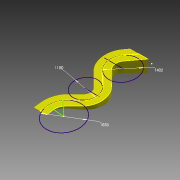
# Autodesk Inventor part: Down Hill_赤2
Saved by Autodesk Inventor 2015 (Build 190159000, 159)
## iProperties
Created: 2015-09-14
Part Number: Down Hill_赤2
Material: 一般
Document SubType Name: Modeling
Designer: nobuhiro
Density: 1 g/cm^3
Appearance: 滑らか - 黄
Author: nobuhiro
Autodesk Inventor part; units mm, degrees
ref_plane "YZ Plane" through (0, 0, 0) normal (1, 0, 0) x (0, 1, 0)
ref_plane "XZ Plane" through (0, 0, 0) normal (0, 1, 0) x (-1, 0, 0)
ref_plane "XY Plane" through (0, 0, 0) normal (0, 0, 1) x (1, 0, 0)
sketch "スケッチ1" plane through (0, 0, 0) normal (0, 0, 1) x (1, 0, 0)
  line L0 (1130.6278, 0) -> (1301.8139, -171.1861)
  line L1 (282.0996, 0) -> (877.5498, -595.4502)
  line L2 (1130.6278, 0) -> (282.0996, 0)
  circle A0 centre (594, -879) radius 1001 construction
  arc A1 (1296.7129, -1591.8784) -> (1296.7129, -1591.8784) centre (389.9346, -671.9826) ccw
  line L3 (1296.7129, -1591.8784) -> (686.4168, -2193.4718)
  circle A2 centre (890, -2400) radius 290 construction
  line L4 (713.3557, -2629.993) -> (1149.395, -2964.8896)
  line L5 (1595, -4169) -> (1595, -3869)
  circle A3 centre (455, -3869) radius 1140 construction
  arc A4 (875.5064, -1164.5786) -> (877.5498, -595.4502) centre (594, -879) ccw construction
  circle A5 centre (890, -2400) radius 890 construction
  circle A6 centre (455, -3869) radius 540 construction
  line L6 (783.9239, -3440.7372) -> (347.8846, -3105.8406)
  line L7 (265.2103, -1766.1721) -> (875.5064, -1164.5786)
  line L8 (995, -3869) -> (995, -4169)
  line L9 (995, -4169) -> (1595, -4169)
  arc A7 (1296.7129, -1591.8784) -> (1301.8139, -171.1861) centre (594, -879) ccw
  arc A8 (265.2103, -1766.1721) -> (347.8846, -3105.8406) centre (890, -2400) ccw
  arc A9 (686.4168, -2193.4718) -> (713.3557, -2629.993) centre (890, -2400) ccw
  arc A10 (875.5064, -1164.5786) -> (877.5498, -595.4502) centre (594, -879) ccw
  arc A11 (995, -3869) -> (783.9239, -3440.7372) centre (455, -3869) ccw
  arc A12 (1595, -3869) -> (1149.395, -2964.8896) centre (455, -3869) ccw
  line L10 (0, -4169) -> (1595, -4169) construction
  line L11 (1595, -4169) -> (1595, -4131.3008) construction
  line L12 (0, -4169) -> (0, 0) construction
  line L13 (0, 0) -> (1595, 0) construction
  line L14 (-1130.6278, 0) -> (-1301.8139, -171.1861)
  line L15 (-282.0996, 0) -> (-877.5498, -595.4502)
  line L16 (-1130.6278, 0) -> (-282.0996, 0)
  arc A13 (-1296.7129, -1591.8784) -> (-1296.7129, -1591.8784) centre (-389.9346, -671.9826) ccw
  line L17 (-1296.7129, -1591.8784) -> (-686.4168, -2193.4718)
  line L18 (-713.3557, -2629.993) -> (-1149.395, -2964.8896)
  line L19 (-1595, -4169) -> (-1595, -3869)
  line L20 (-783.9239, -3440.7372) -> (-347.8846, -3105.8406)
  line L21 (-265.2103, -1766.1721) -> (-875.5064, -1164.5786)
  line L22 (-995, -3869) -> (-995, -4169)
  line L23 (-995, -4169) -> (-1595, -4169)
  arc A14 (-1301.8139, -171.1861) -> (-1296.7129, -1591.8784) centre (-594, -879) ccw
  arc A15 (-347.8846, -3105.8406) -> (-265.2103, -1766.1721) centre (-890, -2400) ccw
  arc A16 (-713.3557, -2629.993) -> (-686.4168, -2193.4718) centre (-890, -2400) ccw
  arc A17 (-877.5498, -595.4502) -> (-875.5064, -1164.5786) centre (-594, -879) ccw
  arc A18 (-783.9239, -3440.7372) -> (-995, -3869) centre (-455, -3869) ccw
  arc A19 (-1149.395, -2964.8896) -> (-1595, -3869) centre (-455, -3869) ccw
  line L24 (0, -4169) -> (-1595, -4169) construction
  line L25 (-1595, -4169) -> (-1595, -4131.3008) construction
  line L26 (1595, -4169) -> (1595, 0) construction
  arc A20 (1120.2352, -2943.2235) -> (532.7643, -2869.5558) centre (890, -2400) ccw
  arc A21 (1086.1097, -1378.2285) -> (1089.6819, -383.3181) centre (594, -879) ccw
  line L27 (332.9203, 373.4434) -> (1089.6819, -383.3181)
  line L28 (475.8136, -1979.822) -> (1086.1097, -1378.2285)
  arc A22 (1295, -3933.8556) -> (965.1205, -3198.4902) centre (455, -3869) ccw
  line L29 (1295, -4169) -> (1295, -3933.8556)
  line L30 (965.1205, -3198.4902) -> (532.7643, -2869.5558)
  dimension "d1" = 1080
  dimension "d2" = 2280
  dimension "d3" = 580
  dimension "d4" = 1780
  dimension "d5" = 802
  dimension "d6" = 2002
  dimension "d16" = 45
  dimension "d19" = 1140
  dimension "d20" = 4169
  dimension "d21" = 0
  dimension "d22" = 600
  dimension "d35" = 3290
  dimension "d36" = 1769
  dimension "d37" = 300
  dimension "d39" = 300
  dimension "d41" = 1595
  dimension "d43" = 1001
  dimension "d55" = 1180
  dimension "d58" = 1402
  dimension "d59" = 300
  dimension "d60" = 1685
  dimension "d61" = 300
  constraints: 62 end point, 49 point on circle, 26 symmetric about line, 23 centre point, 20 tangent, 4 horizontal, 3 coincident, 3 parallel, 2 concentric, 2 perpendicular, 2 point on line, 1 collinear, 1 vertical, 7 other
  measures "d1" diameter of A6
  measures "d2" diameter of A3
  measures "d3" diameter of A2
  measures "d4" diameter of A5
  measures "d5" diameter of A4
  measures "d6" diameter of A0
  measures "d16" angle of L13 L1
  measures "d19" distance from line of A6.centre L11
  measures "d20" distance between parallel lines of L13 L10
  measures "d21" distance between parallel lines of L11 L5
  measures "d22" distance of L8.end L5.start
  measures "d35" distance from line of L10 A0.centre
  measures "d36" distance from line of L10 A5.centre
  measures "d37" distance from line of L10 A3.centre
  measures "d39" distance from line of L10 A6.centre
  measures "d41" distance between parallel lines of L12 L26
  measures "d43" distance from line of L26 A4.centre
  measures "d55" diameter of A20
  measures "d58" diameter of A21
  measures "d59" distance between parallel lines of L27 L1
  measures "d60" diameter of A22
  measures "d61" distance from line of L5.start L29
extrude "押し出し1" add sketch "スケッチ1" along normal blind 600 contours L16 L15 A17 A1 | A1 A17 L21 A15 A13 A14 L14 L16 | A13 A15 L20 A18 L22 L23 L19 A19 L18 A16 L17 | L21 A15 A1
sketch "スケッチ2" plane through (0, 0, 0) normal (1, 0, 0) x (0, 1, 0)
  line L0 (0, 0) -> (0, 600)
  line L1 (0, 600) -> (-4169, 0)
  line L2 (-4169, 0) -> (0, 0)
  dimension "d26" = 600
  dimension "d27" = 4169
  constraints: 6 end point, 1 perpendicular, 1 vertical
  measures "d26" distance of L0.start L0.end
  measures "d27" distance of L1.end L0.start
extrude "押し出し2" cut sketch "スケッチ2" along normal through all both and the other way through all keep common part
sketch "スケッチ3" plane through (-1130.6278, 0, 600) normal (0, -0.1424517, 0.9898018) x (1, 0, 0)
  line L0 (0, 0) -> (-171.1861, -172.9499) projected
  ellipse E0 centre (536.6278, -888.0566) end of major axis (536.6278, 123.257) minor radius 1001 (-171.1861, -172.9499) -> (-166.0851, -1608.28) ccw projected
  line L1 (-166.0851, -1608.28) -> (444.2109, -2216.0718) projected
  ellipse E1 centre (240.6278, -2424.728) end of major axis (240.6278, -2131.74) minor radius 290 (417.2721, -2657.0907) -> (444.2109, -2216.0718) ccw projected
  line L2 (417.2721, -2657.0907) -> (-18.7672, -2995.4378) projected
  ellipse E2 centre (675.6278, -3908.8635) end of major axis (675.6278, -2757.1178) minor radius 1140 (-18.7672, -2995.4378) -> (-464.3722, -3908.8635) ccw projected
  line L3 (-464.3722, -3908.8635) -> (-464.3722, -4211.9545) projected
  line L4 (-464.3722, -4211.9545) -> (135.6278, -4211.9545) projected
  line L5 (135.6278, -4211.9545) -> (135.6278, -3908.8635) projected
  ellipse E3 centre (675.6278, -3908.8635) end of major axis (675.6278, -4454.4273) minor radius 540 (346.7038, -3476.1882) -> (135.6278, -3908.8635) ccw projected
  line L6 (346.7038, -3476.1882) -> (782.7431, -3137.841) projected
  ellipse E4 centre (240.6278, -2424.728) end of major axis (240.6278, -3323.8979) minor radius 890 (782.7431, -3137.841) -> (865.4175, -1784.3695) ccw projected
  line L7 (865.4175, -1784.3695) -> (255.1214, -1176.5777) projected
  ellipse E5 centre (536.6278, -888.0566) end of major axis (536.6278, -1293.1882) minor radius 401 (253.078, -601.5853) -> (255.1214, -1176.5777) ccw projected
  line L8 (253.078, -601.5853) -> (848.5281, 0) projected
  line L9 (848.5281, 0) -> (0, 0) projected
  line L10 (32.4595, -374.5187) -> (119.5473, -286.5336)
  line L11 (119.5473, -286.5336) -> (161.7579, -286.5336)
  line L12 (161.7579, -286.5336) -> (49.4323, -400.0165)
  line L13 (52.9285, -1379.6036) -> (663.2246, -1987.3955)
  line L14 (607.0857, -2911.4653) -> (171.0464, -3249.8125)
  line L15 (-150.9058, -3908.8635) -> (-150.9058, -3925.4209)
  line L16 (-150.9058, -3925.4209) -> (-177.8386, -3925.4209)
  line L17 (-177.8386, -3925.4209) -> (-177.8386, -3908.8635)
  line L18 (156.8903, -3221.8135) -> (592.9296, -2883.4664)
  line L19 (646.4038, -2013.0459) -> (36.1077, -1405.254)
  line L20 (-177.8386, -3925.4209) -> (-177.8386, -4211.9545)
  line L21 (-150.9058, -3925.4209) -> (-150.9058, -4211.9545)
  line L22 (119.5473, -286.5336) -> (403.1588, 0)
  line L23 (161.7579, -286.5336) -> (445.3694, 0)
  line L24 (135.6278, -4196.9545) -> (-464.3722, -4196.9545)
  spline S0 degree 5 poles (49.4323, -400.0165) (6.0772, -443.8184) (-32.3846, -492.4635) (-65.2456, -545.2099) (-132.8167, -686.6868) (-159.1151, -842.5379) (-158.774, -938.5796) (-131.3678, -1094.2411) (-62.7886, -1235.2334) (-29.5508, -1287.7445) (9.2593, -1336.1136) (52.9285, -1379.6037) knots 0 0 0 0 0 0 0.283408 0.283408 0.283408 0.716588 0.716588 0.716588 1 1 1 1 1 1
  spline S1 degree 5 poles (663.2246, -1987.3955) (689.0757, -2013.1406) (712.9955, -2040.8251) (734.7988, -2070.2469) (790.8712, -2159.0366) (827.2909, -2258.2936) (841.914, -2325.8413) (852.2743, -2463.1111) (825.3116, -2598.1007) (802.6182, -2663.2752) (754.4609, -2757.1689) (688.0629, -2838.2566) (662.8873, -2864.7026) (635.8251, -2889.1648) (607.0856, -2911.4653) knots 0 0 0 0 0 0 0.174362 0.174362 0.174362 0.5005 0.5005 0.5005 0.826151 0.826151 0.826151 1 1 1 1 1 1
  spline S2 degree 5 poles (171.0463, -3249.8125) (111.0424, -3296.3728) (56.3825, -3349.8197) (8.1044, -3409.3151) (-74.0223, -3538.2511) (-125.0897, -3682.3398) (-142.3005, -3756.981) (-150.9059, -3832.9223) (-150.9059, -3908.8635) knots 0 0 0 0 0 0 0.500027 0.500027 0.500027 1 1 1 1 1 1
  spline S3 degree 5 poles (-177.8386, -3908.8635) (-177.8386, -3829.4629) (-168.8535, -3750.0621) (-150.8837, -3672.0169) (-97.7184, -3521.8667) (-12.2191, -3387.4922) (37.8624, -3325.6829) (94.5891, -3270.1564) (156.8903, -3221.8135) knots 0 0 0 0 0 0 0.501717 0.501717 0.501717 1 1 1 1 1 1
  spline S4 degree 5 poles (592.9296, -2883.4664) (637.1161, -2849.1796) (677.1472, -2809.5378) (712.1687, -2765.2259) (786.2835, -2643.7028) (821.3073, -2504.3486) (826.6322, -2417.1494) (808.8484, -2274.6041) (750.1598, -2144.9634) (720.8492, -2096.7232) (686.0109, -2052.4905) (646.4039, -2013.0458) knots 0 0 0 0 0 0 0.283586 0.283586 0.283586 0.71657 0.71657 0.71657 1 1 1 1 1 1
  spline S5 degree 5 poles (36.1078, -1405.254) (7.8648, -1377.1269) (-18.4304, -1347.0438) (-42.6049, -1315.1925) (-105.4626, -1219.3372) (-148.7354, -1112.4732) (-167.8679, -1039.6342) (-187.2712, -890.6974) (-168.9256, -741.6264) (-150.3095, -668.6481) (-107.7943, -561.4682) (-45.6173, -465.1561) (-21.6678, -433.1277) (4.4149, -402.8522) (32.4595, -374.5187) knots 0 0 0 0 0 0 0.174265 0.174265 0.174265 0.499975 0.499975 0.499975 0.825708 0.825708 0.825708 1 1 1 1 1 1
  point P0 (1130.6278, -85.471)
  dimension "d31" = 30
  dimension "d32" = 15
  constraints: 30 end point, 11 parallel, 6 point on line, 2 collinear, 2 perpendicular, 1 vertical, 28 other
  measures "d31" distance between parallel lines of L12 L10
  measures "d32" distance between parallel lines of L4 L24
extrude "押し出し3" add sketch "スケッチ3" along normal blind 0.1 contours L9 L23 L11 L22 | L11 L12 S0 L13 S1 L14 S2 L15 L16 L17 S3 L18 S4 L19 S5 L10 | L24 L21 L4 L20 | L20 L16 L21 L24
sketch "スケッチ5" plane through (0, 0, 0) normal (0, 0, 1) x (1, 0, 0)
  line L0 (-1308.4664, -3869.0142) -> (-1308.4664, -4169.0142) projected
  line L1 (-1308.4664, -4169.0142) -> (-1281.5336, -4169.0142) projected
  line L2 (-1281.5336, -4169.0142) -> (-1281.5336, -3869.0142) projected
  line L3 (-959.5814, -3216.6844) -> (-523.5421, -2881.7878) projected
  line L4 (-467.4032, -1967.1418) -> (-1077.6993, -1365.5484) projected
  line L5 (-1081.1954, -395.9513) -> (-685.2584, -0.0142) projected
  line L6 (-685.2584, -0.0142) -> (-727.469, -0.0142) projected
  line L7 (-727.469, -0.0142) -> (-1098.1683, -370.7135) projected
  line L8 (-1094.52, -1390.9371) -> (-484.2239, -1992.5306) projected
  line L9 (-537.6982, -2854.0743) -> (-973.7375, -3188.9709) projected
  line L10 (-1081.1954, -395.9513) -> (-598.1176, -879.0291)
  line L11 (-598.1176, -879.0291) -> (-1077.6993, -1365.5484)
  line L12 (-598.1176, -879.0291) -> (-1281.5292, -881.4829)
  line L13 (-1281.5292, -881.4829) -> (-1308.4618, -881.5796)
  line L14 (-484.2239, -1992.5306) -> (-886.1997, -2400.3213)
  line L15 (-886.1997, -2400.3213) -> (-537.6982, -2854.0743)
  line L16 (-886.1997, -2400.3213) -> (-314.5767, -2435.5976)
  line L17 (-314.5767, -2435.5976) -> (-287.673, -2437.2579)
  line L18 (-1281.5336, -3869.0142) -> (-458.5645, -3869.0142)
  line L19 (-458.5645, -3869.0142) -> (-959.5814, -3216.6844)
  line L20 (-458.5645, -3869.0142) -> (-1196.5639, -3505.2796)
  line L21 (-1196.5639, -3505.2796) -> (-1221.7346, -3492.8739)
  point P0 (0, 0)
  point P1 (-1294.9955, -881.5312)
  point P2 (-301.1248, -2436.4277)
  point P3 (-1209.1492, -3499.0768)
  point P4 (536.9761, 8076.7198)
  dimension "d44" = 669.9375
  dimension "d45" = 1732.5865
  dimension "d46" = 3287.483
  constraints: 24 end point, 3 collinear, 3 midpoint, 1 horizontal, 20 other
  measures "d44" distance from line of L1 point (-1209.149, -3499.077)
  measures "d45" distance from line of L1 point (-301.125, -2436.428)
  measures "d46" distance from line of point (-1294.995, -881.531) L1
sketch "スケッチ6" plane through (0, 0, 0) normal (1, 0, 0) x (0, 1, 0)
  line L0 (-3869.0142, 43.2748) -> (-4169.0142, 0.099) projected
  line L1 (-4169.0142, 0.099) -> (-3869.0142, 43.2748) projected
  line L2 (-3869.0142, 43.2748) -> (-3216.6844, 137.1577) projected
  line L3 (-3216.6844, 137.1577) -> (-2881.7878, 185.3559) projected
  line L4 (-2881.7878, 185.3559) -> (-1967.1418, 316.9912) projected
  line L5 (-1967.1418, 316.9912) -> (-1365.5484, 403.5721) projected
  line L6 (-1365.5484, 403.5721) -> (-395.9513, 543.116) projected
  line L7 (-395.9513, 543.116) -> (-0.0142, 600.099) projected
  line L8 (-0.0142, 600.099) -> (-370.7135, 546.7482) projected
  line L9 (-370.7135, 546.7482) -> (-1390.9371, 399.9182) projected
  line L10 (-1390.9371, 399.9182) -> (-1992.5306, 313.3372) projected
  line L11 (-1992.5306, 313.3372) -> (-2854.0743, 189.3444) projected
  line L12 (-2854.0743, 189.3444) -> (-3188.9709, 141.1462) projected
  line L13 (-3188.9709, 141.1462) -> (-3869.0142, 43.2748) projected
  point P0 (0, 0)
  point P1 (-3499.0768, 96.516)
  point P2 (-2436.4277, 249.4518)
  point P3 (-881.5312, 473.2316)
  dimension "d47" = 669.9375
  dimension "d48" = 1732.5865
  dimension "d49" = 3287.483
  dimension "d50" = 96.417
  dimension "d51" = 249.3528
  dimension "d52" = 473.1326
  constraints: 3 point on line
  measures "d47" horizontal distance of point (-3499.077, 96.516) L0.end
  measures "d48" horizontal distance of L0.end point (-2436.428, 249.452)
  measures "d49" horizontal distance of L0.end point (-881.531, 473.232)
  measures "d50" vertical distance of point (-3499.077, 96.516) L0.end
  measures "d51" vertical distance of L0.end point (-2436.428, 249.452)
  measures "d52" vertical distance of L0.end point (-881.531, 473.232)
sketch "スケッチ7" plane through (-1130.6278, -0.0142, 600.099) normal (0, -0.1424517, 0.9898018) x (1, 0, 0)
  line L0 (-177.8386, -3908.8635) -> (-177.8386, -4211.9545) projected
  line L1 (-177.8386, -4211.9545) -> (-150.9058, -4211.9545) projected
  line L2 (-150.9058, -4211.9545) -> (-150.9058, -3908.8635) projected
  line L3 (171.0464, -3249.8125) -> (607.0857, -2911.4653) projected
  line L4 (663.2246, -1987.3955) -> (52.9285, -1379.6036) projected
  line L5 (49.4323, -400.0165) -> (445.3694, 0) projected
  line L6 (445.3694, 0) -> (403.1588, 0) projected
  line L7 (403.1588, 0) -> (32.4595, -374.5187) projected
  line L8 (36.1077, -1405.254) -> (646.4038, -2013.0459) projected
  line L9 (592.9296, -2883.4664) -> (156.8903, -3221.8135) projected
  line L10 (-150.9058, -3908.8635) -> (-150.9058, -4211.9545) projected
  line L11 (-150.9058, -4211.9545) -> (135.6278, -4211.9545) projected
  line L12 (135.6278, -4211.9545) -> (135.6278, -3908.8635) projected
  ellipse E0 centre (675.6278, -3908.8635) end of major axis (675.6278, -4454.4273) minor radius 540 (346.7038, -3476.1882) -> (135.6278, -3908.8635) ccw projected
  line L13 (346.7038, -3476.1882) -> (782.7431, -3137.841) projected
  ellipse E1 centre (240.6278, -2424.728) end of major axis (240.6278, -3323.8979) minor radius 890 (782.7431, -3137.841) -> (865.4175, -1784.3695) ccw projected
  line L14 (865.4175, -1784.3695) -> (255.1214, -1176.5777) projected
  ellipse E2 centre (536.6278, -888.0566) end of major axis (536.6278, -1293.1882) minor radius 401 (253.078, -601.5853) -> (255.1214, -1176.5777) ccw projected
  line L15 (253.078, -601.5853) -> (848.5281, 0) projected
  line L16 (848.5281, 0) -> (445.3694, 0) projected
  line L17 (445.3694, 0) -> (49.4323, -400.0165) projected
  line L18 (52.9285, -1379.6036) -> (663.2246, -1987.3955) projected
  line L19 (607.0857, -2911.4653) -> (171.0464, -3249.8125) projected
  line L20 (536.6278, -888.0566) -> (-363.5747, -888.0566)
  line L21 (240.6278, -2424.728) -> (865.4175, -2424.728)
  circle A0 centre (675.6278, -3908.8635) radius 842.5
  circle A1 centre (240.6278, -2424.728) radius 590
  circle A2 centre (536.6278, -888.0566) radius 701
  line L22 (675.6278, -3908.8635) -> (-164.3722, -3844.0079)
  line L23 (675.6278, -3908.8635) -> (52.6201, -3341.706)
  point P0 (1130.6278, -85.471)
  point P1 (-164.3722, -888.0566)
  point P2 (830.6278, -2424.728)
  point P3 (-164.3722, -888.0566)
  point P4 (830.6278, -2424.728)
  dimension "d56" = 1180
  dimension "d57" = 1402
  dimension "d54" = 1685
  constraints: 8 end point, 6 coincident, 2 horizontal, 2 horizontal alignment, 2 point on circle, 2 point on line, 1 centre point, 16 other
  measures "d54" diameter of A0
equation "\"d47\" = d44"
equation "\"d48\" = d45"
equation "\"d49\" = d46"
